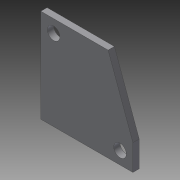
# Autodesk Inventor part: top_plate
Saved by Autodesk Inventor 2015 (Build 190159000, 159)
## iProperties
Created: 2015-06-21
Part Number: top_plate
Material: Generic
Document SubType Name: Modeling
Designer: Master
Density: 1 g/cm^3
Appearance: Default
Author: Master
Autodesk Inventor part; units mm, degrees
ref_plane "YZ Plane" through (0, 0, 0) normal (1, 0, 0) x (0, 1, 0)
ref_plane "XZ Plane" through (0, 0, 0) normal (0, 1, 0) x (-1, 0, 0)
ref_plane "XY Plane" through (0, 0, 0) normal (0, 0, 1) x (1, 0, 0)
sketch "Sketch1" plane through (0, 0, 0) normal (0, 0, 1) x (1, 0, 0)
  line L0 (3, -6) -> (-3, -6) projected
  line L1 (3, 21) -> (3, -6) projected
  line L2 (-3, 21) -> (3, 21) projected
  line L3 (-3, -6) -> (-3, 21) projected
  circle A0 centre (15.8383, 17.8821) radius 1.5 projected
  line L4 (18.8902, -6) -> (18.8902, 21) projected
  line L5 (13, 21) -> (18.8902, 21) projected
  line L6 (13, -6) -> (13, 21) projected
  line L7 (18.8902, -6) -> (13, -6) projected
  circle A1 centre (0.0519, 34.1179) radius 1.5 projected
  line L8 (3, 46) -> (3, 31) projected
  line L9 (-3, 46) -> (3, 46) projected
  line L10 (-3, 31) -> (-3, 46) projected
  line L11 (3, 31) -> (-3, 31) projected
  line L12 (18.8902, 14.8821) -> (-3, 14.8821)
  line L13 (-3, 14.8821) -> (-3, 37.1179)
  line L14 (-3, 37.1179) -> (13, 37.1179)
  line L15 (18.8902, 21) -> (18.8902, 14.8821)
  line L16 (18.8902, 21) -> (13, 37.1179)
  point P0 (0, 0)
  dimension "d0" = 3
  dimension "d1" = 3
  constraints: 10 end point, 4 point on line
  measures "d0" distance from line of L12 A0.centre
  measures "d1" distance from line of A1.centre L14
extrude "Extrusion1" add sketch "Sketch1" along normal blind 1.5 contours L12 L3 L2 L1 | L1 L2 L13 L11 L8 L14 L16 L5 L6 L12 | L6 L5 L4 L12 | L10 L14 L8 L11
body "Solid1"
